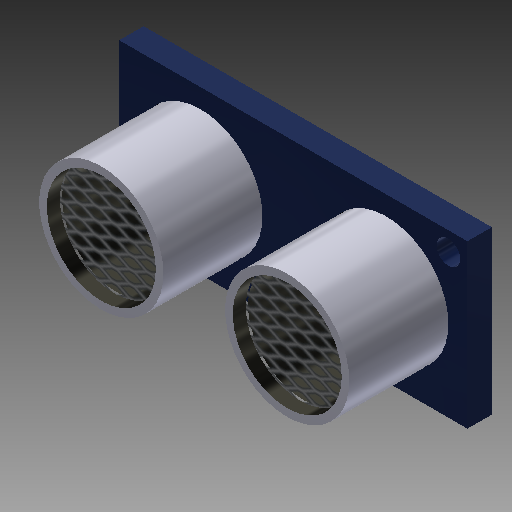
# Autodesk Inventor part: ping
Saved by Autodesk Inventor 2018.3 (Build 223284000, 284)
## iProperties
Created: 2015-07-03
Part Number: ping
Material: 一般
Document SubType Name: Modeling
Designer: Shinichi
Density: 1 g/cm^3
Appearance: 既定
Mass: 3.01792 g
Surface Area: 61.3471 cm^2
Volume: 3.01792 cm^3
Author: Shinichi
Autodesk Inventor part; units mm, degrees
ref_plane "YZ Plane" through (0, 0, 0) normal (1, 0, 0) x (0, 1, 0)
ref_plane "XZ Plane" through (0, 0, 0) normal (0, 1, 0) x (-1, 0, 0)
sketch "スケッチ1" plane through (0, 0, 0) normal (0, 0, 1) x (1, 0, 0)
  line L0 (22.85, 13.15) -> (-22.85, 13.15)
  line L1 (-22.85, 13.15) -> (-22.85, -8.15)
  line L2 (-22.85, -8.15) -> (22.85, -8.15)
  line L3 (22.85, -8.15) -> (22.85, 13.15)
  circle A0 centre (20.35, 10.65) radius 1.55
  circle A1 centre (-20.35, -5.65) radius 1.55
  circle A2 centre (12.2, 2.5) radius 8.15
  circle A3 centre (-12.2, 2.5) radius 8.15
  line L4 (-2.5, -13.15) -> (-2.5, -8.15)
  line L5 (0, -8.15) -> (0, -13.15)
  line L6 (2.5, -13.15) -> (2.5, -8.15)
  point P0 (0, 0)
  constraints: 14 end point, 5 perpendicular, 4 centre point, 2 equal radius, 2 point on line, 1 midpoint, 1 parallel
extrude "押し出し1" add sketch "スケッチ1" along normal blind 3.2 contours L3 L2 L1 L0 | A2 | A3
sketch "スケッチ2" plane through (0, 0, 3.2) normal (0, 0, 1) x (1, 0, 0)
  line L0 (22.85, 13.15) -> (-22.85, 13.15)
  line L1 (-22.85, 13.15) -> (-22.85, -8.15)
  line L2 (-22.85, -8.15) -> (22.85, -8.15)
  line L3 (22.85, -8.15) -> (22.85, 13.15)
  circle A0 centre (20.35, 10.65) radius 1.55
  circle A1 centre (-20.35, -5.65) radius 1.55
  circle A2 centre (12.2, 2.5) radius 8.15
  circle A3 centre (-12.2, 2.5) radius 8.15
  line L4 (-2.5, -13.15) -> (-2.5, -8.15)
  line L5 (0, -8.15) -> (0, -13.15)
  line L6 (2.5, -13.15) -> (2.5, -8.15)
  point P0 (0, 0)
  constraints: 14 end point, 5 perpendicular, 4 centre point, 2 equal radius, 2 point on line, 1 midpoint, 1 parallel
extrude "押し出し2" add sketch "スケッチ2" along normal blind 13 contours A2 | A3
shell "シェル1" thickness 1 removed faces 2 at (-11.3117, 0.2642, 16.2) at (12.9427, 4.4582, 16.2)
ref_plane "作業平面2" through (0, 0, 14.2) normal (0, 0, 1) x (1, 0, 0)
sketch "スケッチ6" plane through (0, 0, 14.2) normal (0, 0, 1) x (1, 0, 0)
  circle A0 centre (-12.2, 2.5) radius 7.15 projected
  line L0 (-19.35, 2.5) -> (-5.05, 2.5)
  circle A1 centre (-12.2, 2.5) radius 7.15
  line L1 (-19.052, 4.5426) -> (-5.3543, 4.5637)
  line L2 (-18.3489, 6.1487) -> (-5.9959, 6.0541)
  line L3 (-17.2114, 7.5999) -> (-7.2004, 7.6115)
  line L4 (-19.1499, 0.8202) -> (-5.2376, 0.8727)
  line L5 (-18.534, -0.8171) -> (-5.6692, -0.4105)
  line L6 (-17.3855, -2.4227) -> (-7.0375, -2.4468)
  line L7 (-16.0004, -3.5563) -> (-8.3492, -3.5245)
  line L8 (-17.2114, 7.5999) -> (-17.3855, -2.4227)
  line L9 (-14.4249, 9.295) -> (-14.3135, -4.3305)
  line L10 (-13.1954, 9.5804) -> (-13.1455, -4.5872)
  line L11 (-11.4954, 9.6152) -> (-11.3318, -4.5971)
  line L12 (-12.4363, 9.6461) -> (-12.1311, -4.6497)
  line L13 (-10.5067, 9.4466) -> (-10.5519, -4.4575)
  line L14 (-9.4473, 9.0989) -> (-9.235, -4.0063)
  line L15 (-8.5464, 8.646) -> (-8.3492, -3.5245)
  line L16 (-7.2004, 7.6115) -> (-7.0375, -2.4468)
  line L17 (-6.2491, 6.4635) -> (-6.0315, -0.4219)
  line L18 (-5.3543, 4.5637) -> (-5.2376, 0.8727)
  line L19 (-16.2779, 8.3731) -> (-16.2973, -3.3596)
  line L20 (-15.5086, 8.8384) -> (-15.311, -3.9377)
  line L21 (-15.5086, 8.8384) -> (-8.1551, 8.3959)
  line L22 (-19.2523, 3.678) -> (-5.1166, 3.4733)
  line L23 (-19.2938, 1.605) -> (-5.0932, 1.7148)
  line L24 (-18.0596, 6.5972) -> (-18.2101, -1.3732)
  line L25 (-18.8956, -0.0083) -> (-5.4358, 0.183)
  line L26 (-17.9612, -1.7345) -> (-6.2041, -1.3951)
  line L27 (-6.0315, -0.4219) -> (-6.2041, -1.3951)
  point P0 (0, 0)
  constraints: 56 end point, 3 parallel, 1 coincident, 1 horizontal, 1 perpendicular, 1 point on line, 91 other
sketch "スケッチ7" plane through (0, 0, 14.2) normal (0, 0, 1) x (1, 0, 0)
  circle A0 centre (-12.2, 2.5) radius 7.15 projected
  line L0 (-19.35, 2.5) -> (-12.2, 2.5)
  circle A1 centre (-12.2, 2.5) radius 7.15
  circle A2 centre (12.2, 2.5) radius 7.15 projected
  line L1 (5.05, 2.5) -> (12.2, 2.5)
  circle A3 centre (12.2, 2.5) radius 7.15
  point P0 (0, 0)
  constraints: 4 end point, 2 centre point, 2 coincident, 2 horizontal, 2 horizontal alignment, 4 other
sketch "スケッチ8" plane through (0, 0, 3.2) normal (0, 0, 1) x (1, 0, 0)
  circle A0 centre (-12.1996, 2.4988) radius 2.8
  circle A1 centre (12.2866, 2.4988) radius 2.8
  point P0 (0, 0)
  dimension "d8" = 5.6
  dimension "d9" = 5.6
  constraints: 2 centre point
  measures "d8" diameter of A0
  measures "d9" diameter of A1
extrude "押し出し4" add sketch "スケッチ8" along normal blind 3
extrude "押し出し5" add sketch "スケッチ7" along normal blind 0.3
